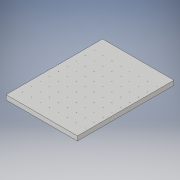
# Autodesk Inventor part: Gantry Base
Saved by Autodesk Inventor 2019.4 (Build 234330000, 330)
## iProperties
Created: 2021-01-12
Part Number: Gantry Base
Material: Generic
Document SubType Name: Modeling
Designer: caleb
Density: 1 g/cm^3
Appearance: Default
Author: caleb
Autodesk Inventor part; units mm, degrees
ref_plane "YZ Plane" through (0, 0, 0) normal (1, 0, 0) x (0, 1, 0)
ref_plane "XZ Plane" through (0, 0, 0) normal (0, 1, 0) x (-1, 0, 0)
ref_plane "XY Plane" through (0, 0, 0) normal (0, 0, 1) x (1, 0, 0)
sketch "Sketch1" plane through (0, 0, 0) normal (0, 1, 0) x (-1, 0, 0)
  line L0 (-609.6, 823.468) -> (609.6, 823.468)
  line L1 (609.6, 823.468) -> (609.6, -823.468)
  line L2 (609.6, -823.468) -> (-609.6, -823.468)
  line L3 (-609.6, -823.468) -> (-609.6, 823.468)
  line L4 (-609.6, 823.468) -> (609.6, -823.468) construction
  line L5 (609.6, 823.468) -> (-609.6, -823.468) construction
  point P0 (0, 0)
  dimension "d0" = 1219.2
  dimension "d1" = 1646.936
  constraints: 12 end point, 2 midpoint, 2 parallel, 1 horizontal, 1 perpendicular
  measures "d0" distance of L0.start L0.end
  measures "d1" distance of L0.end L1.end
extrude "Extrusion1" add sketch "Sketch1" along normal blind 76.2
sketch "Sketch2" plane through (0, 76.2, 0) normal (0, 1, 0) x (1, 0, 0)
  circle A0 centre (558.8, -641.35) radius 3.175
  line L0 (-609.6, -823.468) -> (609.6, -823.468) projected
  line L1 (609.6, -823.468) -> (609.6, 823.468) projected
  circle A1 centre (558.8, -488.95) radius 3.175
  circle A2 centre (558.8, -336.55) radius 3.175
  circle A3 centre (558.8, -184.15) radius 3.175
  circle A4 centre (558.8, -31.75) radius 3.175
  circle A5 centre (558.8, 120.65) radius 3.175
  circle A6 centre (558.8, 273.05) radius 3.175
  circle A7 centre (558.8, 425.45) radius 3.175
  circle A8 centre (558.8, 577.85) radius 3.175
  circle A9 centre (406.4, -641.35) radius 3.175
  circle A10 centre (406.4, -488.95) radius 3.175
  circle A11 centre (406.4, -336.55) radius 3.175
  circle A12 centre (406.4, -184.15) radius 3.175
  circle A13 centre (406.4, -31.75) radius 3.175
  circle A14 centre (406.4, 120.65) radius 3.175
  circle A15 centre (406.4, 273.05) radius 3.175
  circle A16 centre (406.4, 425.45) radius 3.175
  circle A17 centre (406.4, 577.85) radius 3.175
  circle A18 centre (254, -641.35) radius 3.175
  circle A19 centre (254, -488.95) radius 3.175
  circle A20 centre (254, -336.55) radius 3.175
  circle A21 centre (254, -184.15) radius 3.175
  circle A22 centre (254, -31.75) radius 3.175
  circle A23 centre (254, 120.65) radius 3.175
  circle A24 centre (254, 273.05) radius 3.175
  circle A25 centre (254, 425.45) radius 3.175
  circle A26 centre (254, 577.85) radius 3.175
  circle A27 centre (101.6, -641.35) radius 3.175
  circle A28 centre (101.6, -488.95) radius 3.175
  circle A29 centre (101.6, -336.55) radius 3.175
  circle A30 centre (101.6, -184.15) radius 3.175
  circle A31 centre (101.6, -31.75) radius 3.175
  circle A32 centre (101.6, 120.65) radius 3.175
  circle A33 centre (101.6, 273.05) radius 3.175
  circle A34 centre (101.6, 425.45) radius 3.175
  circle A35 centre (101.6, 577.85) radius 3.175
  circle A36 centre (-50.8, -641.35) radius 3.175
  circle A37 centre (-50.8, -488.95) radius 3.175
  circle A38 centre (-50.8, -336.55) radius 3.175
  circle A39 centre (-50.8, -184.15) radius 3.175
  circle A40 centre (-50.8, -31.75) radius 3.175
  circle A41 centre (-50.8, 120.65) radius 3.175
  circle A42 centre (-50.8, 273.05) radius 3.175
  circle A43 centre (-50.8, 425.45) radius 3.175
  circle A44 centre (-50.8, 577.85) radius 3.175
  circle A45 centre (-203.2, -641.35) radius 3.175
  circle A46 centre (-203.2, -488.95) radius 3.175
  circle A47 centre (-203.2, -336.55) radius 3.175
  circle A48 centre (-203.2, -184.15) radius 3.175
  circle A49 centre (-203.2, -31.75) radius 3.175
  circle A50 centre (-203.2, 120.65) radius 3.175
  circle A51 centre (-203.2, 273.05) radius 3.175
  circle A52 centre (-203.2, 425.45) radius 3.175
  circle A53 centre (-203.2, 577.85) radius 3.175
  circle A54 centre (-355.6, -641.35) radius 3.175
  circle A55 centre (-355.6, -488.95) radius 3.175
  circle A56 centre (-355.6, -336.55) radius 3.175
  circle A57 centre (-355.6, -184.15) radius 3.175
  circle A58 centre (-355.6, -31.75) radius 3.175
  circle A59 centre (-355.6, 120.65) radius 3.175
  circle A60 centre (-355.6, 273.05) radius 3.175
  circle A61 centre (-355.6, 425.45) radius 3.175
  circle A62 centre (-355.6, 577.85) radius 3.175
  circle A63 centre (-508, -641.35) radius 3.175
  circle A64 centre (-508, -488.95) radius 3.175
  circle A65 centre (-508, -336.55) radius 3.175
  circle A66 centre (-508, -184.15) radius 3.175
  circle A67 centre (-508, -31.75) radius 3.175
  circle A68 centre (-508, 120.65) radius 3.175
  circle A69 centre (-508, 273.05) radius 3.175
  circle A70 centre (-508, 425.45) radius 3.175
  circle A71 centre (-508, 577.85) radius 3.175
  point P0 (0, 0)
  point P1 (-203.2, -184.15)
  dimension "d4" = 6.35
  dimension "d5" = 182.118
  dimension "d6" = 50.8
  dimension "d9" = 152.4
  dimension "d12" = 152.4
  constraints: 72 centre point, 1 coincident, 1 horizontal, 1 vertical, 142 other
  measures "d4" diameter of A0
  measures "d5" distance from line of A0.centre L0
  measures "d6" distance from line of L1 A0.centre
  measures "d9" distance of A0.centre A1.centre
  measures "d12" distance of A0.centre A9.centre
hole "Hole1" at (558.8, 76.2, 641.35) at (558.8, 76.2, 488.95) at (558.8, 76.2, 336.55) at (558.8, 76.2, 184.15) at (558.8, 76.2, 31.75) at (558.8, 76.2, -120.65) at (558.8, 76.2, -273.05) at (558.8, 76.2, -425.45) at (558.8, 76.2, -577.85) at (406.4, 76.2, -577.85) at (406.4, 76.2, -425.45) at (406.4, 76.2, -273.05) at (406.4, 76.2, -120.65) at (406.4, 76.2, 31.75) at (406.4, 76.2, 184.15) at (406.4, 76.2, 336.55) at (406.4, 76.2, 488.95) at (406.4, 76.2, 641.35) at (254, 76.2, 641.35) at (254, 76.2, 488.95) at (254, 76.2, 336.55) at (254, 76.2, 184.15) at (254, 76.2, 31.75) at (254, 76.2, -120.65) at (254, 76.2, -273.05) at (254, 76.2, -425.45) at (254, 76.2, -577.85) at (101.6, 76.2, -577.85) at (101.6, 76.2, -425.45) at (101.6, 76.2, -273.05) at (101.6, 76.2, -120.65) at (101.6, 76.2, 31.75) at (101.6, 76.2, 184.15) at (101.6, 76.2, 336.55) at (101.6, 76.2, 488.95) at (101.6, 76.2, 641.35) at (-50.8, 76.2, 641.35) at (-50.8, 76.2, 488.95) at (-50.8, 76.2, 336.55) at (-50.8, 76.2, 184.15) at (-50.8, 76.2, 31.75) at (-50.8, 76.2, -120.65) at (-50.8, 76.2, -273.05) at (-50.8, 76.2, -425.45) at (-50.8, 76.2, -577.85) at (-203.2, 76.2, -577.85) at (-355.6, 76.2, -577.85) at (-355.6, 76.2, -425.45) at (-203.2, 76.2, -425.45) at (-203.2, 76.2, -273.05) direction (0, -1, 0) diameter 4.9784 end through all and at (-355.6, 76.2, -273.05) (-203.2, 76.2, -120.65) (-203.2, 76.2, 31.75) (-203.2, 76.2, 336.55) (-203.2, 76.2, 488.95) (-203.2, 76.2, 641.35) (-355.6, 76.2, 641.35) (-508, 76.2, 641.35) (-508, 76.2, 488.95) (-355.6, 76.2, 488.95) (-355.6, 76.2, 336.55) (-508, 76.2, 336.55) (-355.6, 76.2, 184.15) (-508, 76.2, 184.15) (-355.6, 76.2, 31.75) (-508, 76.2, 31.75) (-508, 76.2, -120.65) (-355.6, 76.2, -120.65) (-508, 76.2, -273.05) (-508, 76.2, -425.45) (-508, 76.2, -577.85) (-203.2, 76.2, 184.15) thread size "1/4-20 UNC" class "2B" standard "ANSI Unified Screw Threads"
body "Solid1"
